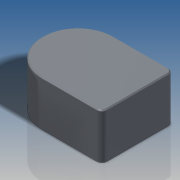
# Autodesk Inventor part: 99145-LtBluishGray
Saved by Autodesk Inventor 2016 SP2 (Build 200236200, 236)
## iProperties
Created: 2015-08-19
Part Number: 99145-LtBluishGray
Material: ABS Plastic
Document SubType Name: Modeling
Designer: D. Kohfeld
Mass: 0.448868 g
Surface Area: 3.37676 cm^2
Volume: 0.423461 cm^3
Density: 1.06 g/cm^3
Appearance: LtBluishGray
Author: D. Kohfeld
Autodesk Inventor part; units mm, degrees
ref_plane "YZ Plane" through (0, 0, 0) normal (1, 0, 0) x (0, 1, 0)
ref_plane "XZ Plane" through (0, 0, 0) normal (0, 1, 0) x (-1, 0, 0)
ref_plane "XY Plane" through (0, 0, 0) normal (0, 0, 1) x (1, 0, 0)
sketch "Sketch2" plane through (0, 0, 0) normal (0, 1, 0) x (-1, 0, 0)
  line L0 (-6.8, 4.08) -> (-6.8, -4.08)
  line L1 (-6.8, -4.08) -> (0, -4.08)
  arc A0 (0, -4.08) -> (0, 4.08) centre (0, 0) ccw
  line L2 (0, 4.08) -> (-6.8, 4.08)
  dimension "d0" = 8.16
  dimension "d1" = 6.8
  constraints: 6 end point, 2 horizontal, 2 point on circle, 2 tangent, 1 centre point, 1 coincident, 1 vertical
  measures "d0" distance between parallel lines of L1 L2
  measures "d1" distance from line of point (0, 0) L0
extrude "Extrusion1" add sketch "Sketch2" along normal mid plane 5.2
fillet "Fillet1" radius 0.6 2 edges at (6.8, 0, 4.08) (6.8, 0, -4.08)
chamfer "Chamfer1" distance 0.12 angle 45 6 edges at (-4.08, 2.6, 0) (3.1, 2.6, 4.08) (6.6243, 2.6, 3.9043) (6.8, 2.6, 0) (6.6243, 2.6, -3.9043) (3.1, 2.6, -4.08)
body "Solid1"
